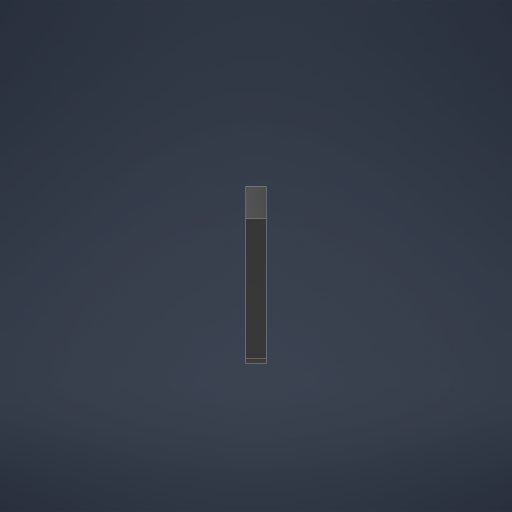
# Autodesk Inventor part: CarbonConnectorStab
Saved by Autodesk Inventor 2023 (Build 270158000, 158)
## iProperties
Created: 2023-02-24
Part Number: CarbonConnectorStab
Material: Generic
Document SubType Name: Modeling
Designer: Elias Braun
Density: 1 g/cm^3
Appearance: Glossy - Black
Author: Elias Braun
Autodesk Inventor part; units mm, degrees
ref_plane "YZ Plane" through (0, 0, 0) normal (1, 0, 0) x (0, 1, 0)
ref_plane "XZ Plane" through (0, 0, 0) normal (0, 1, 0) x (-1, 0, 0)
ref_plane "XY Plane" through (0, 0, 0) normal (0, 0, 1) x (1, 0, 0)
sketch "Sketch3" plane through (0, 0, 0) normal (0, 1, 0) x (-1, 0, 0)
  circle A0 centre (0, 0) radius 110 construction
  arc A1 (43.0581, -98.5) -> (-43.0581, -98.5) centre (0, 0) ccw
  line L0 (0, -107.5) -> (0, -98.5) construction
  line L1 (0, -98.5) -> (0, -73.5) construction
  line L2 (0, -98.5) -> (-43.0581, -98.5) construction
  line L3 (0, -98.5) -> (43.0581, -98.5) construction
  line L4 (43.0581, -98.5) -> (-43.0581, -98.5) construction
  line L5 (-18.0581, -73.5) -> (18.0581, -73.5)
  arc A2 (43.0581, -98.5) -> (18.0581, -73.5) centre (18.0581, -98.5) ccw
  arc A3 (-18.0581, -73.5) -> (-43.0581, -98.5) centre (-18.0581, -98.5) ccw
  line L6 (0, 107.5) -> (0, 97.5) construction
  line L7 (0, 97.5) -> (-22.5, 97.5) construction
  line L8 (-22.5, 97.5) -> (-22.5, 82.5) construction
  line L9 (22.5, 82.5) -> (22.5, 97.5) construction
  line L10 (22.5, 90) -> (-22.5, 90) construction
  line L11 (15, 97.5) -> (-15, 97.5)
  line L12 (-15, 82.5) -> (15, 82.5)
  arc A4 (15, 82.5) -> (15, 97.5) centre (15, 90) ccw
  arc A5 (-15, 97.5) -> (-15, 82.5) centre (-15, 90) ccw
  line L13 (22.5, 82.5) -> (17.5, 82.5) construction
  line L14 (17.5, 82.5) -> (17.5, 77.5) construction
  circle A6 centre (17.5, 77.5) radius 1.6
  circle A7 centre (-17.5, 77.5) radius 1.6
  line L15 (-58.3363, 79.5495) -> (-79.5495, 58.3363)
  arc A8 (-47.7297, 68.9429) -> (-58.3363, 79.5495) centre (-53.033, 74.2462) ccw
  arc A9 (-79.5495, 58.3363) -> (-68.9429, 47.7297) centre (-74.2462, 53.033) ccw
  line L16 (-68.9429, 47.7297) -> (-47.7297, 68.9429)
  circle A10 centre (-67.1751, 42.4264) radius 1.6
  circle A11 centre (-42.4264, 67.1751) radius 1.6
  line L17 (-97.5, 15) -> (-97.5, -15)
  arc A12 (-82.5, 15) -> (-97.5, 15) centre (-90, 15) ccw
  arc A13 (-97.5, -15) -> (-82.5, -15) centre (-90, -15) ccw
  line L18 (-82.5, -15) -> (-82.5, 15)
  circle A14 centre (-77.5, -17.5) radius 1.6
  circle A15 centre (-77.5, 17.5) radius 1.6
  line L19 (-79.5495, -58.3363) -> (-58.3363, -79.5495)
  arc A16 (-68.9429, -47.7297) -> (-79.5495, -58.3363) centre (-74.2462, -53.033) ccw
  arc A17 (-58.3363, -79.5495) -> (-47.7297, -68.9429) centre (-53.033, -74.2462) ccw
  line L20 (-47.7297, -68.9429) -> (-68.9429, -47.7297)
  circle A18 centre (-42.4264, -67.1751) radius 1.6
  circle A19 centre (-67.1751, -42.4264) radius 1.6
  line L21 (-15, -97.5) -> (15, -97.5)
  arc A20 (-15, -82.5) -> (-15, -97.5) centre (-15, -90) ccw
  arc A21 (15, -97.5) -> (15, -82.5) centre (15, -90) ccw
  line L22 (15, -82.5) -> (-15, -82.5)
  circle A22 centre (17.5, -77.5) radius 1.6
  circle A23 centre (-17.5, -77.5) radius 1.6
  line L23 (58.3363, -79.5495) -> (79.5495, -58.3363)
  arc A24 (47.7297, -68.9429) -> (58.3363, -79.5495) centre (53.033, -74.2462) ccw
  arc A25 (79.5495, -58.3363) -> (68.9429, -47.7297) centre (74.2462, -53.033) ccw
  line L24 (68.9429, -47.7297) -> (47.7297, -68.9429)
  circle A26 centre (67.1751, -42.4264) radius 1.6
  circle A27 centre (42.4264, -67.1751) radius 1.6
  line L25 (97.5, -15) -> (97.5, 15)
  arc A28 (82.5, -15) -> (97.5, -15) centre (90, -15) ccw
  arc A29 (97.5, 15) -> (82.5, 15) centre (90, 15) ccw
  line L26 (82.5, 15) -> (82.5, -15)
  circle A30 centre (77.5, 17.5) radius 1.6
  circle A31 centre (77.5, -17.5) radius 1.6
  line L27 (79.5495, 58.3363) -> (58.3363, 79.5495)
  arc A32 (68.9429, 47.7297) -> (79.5495, 58.3363) centre (74.2462, 53.033) ccw
  arc A33 (58.3363, 79.5495) -> (47.7297, 68.9429) centre (53.033, 74.2462) ccw
  line L28 (47.7297, 68.9429) -> (68.9429, 47.7297)
  circle A34 centre (42.4264, 67.1751) radius 1.6
  circle A35 centre (67.1751, 42.4264) radius 1.6
  circle A36 centre (0, 0) radius 110 construction
  arc A37 (43.0581, -98.5) -> (-43.0581, -98.5) centre (0, 0) ccw
  line L29 (0, -107.5) -> (0, -98.5) construction
  line L30 (0, -98.5) -> (0, -73.5) construction
  line L31 (0, -98.5) -> (-43.0581, -98.5) construction
  line L32 (0, -98.5) -> (43.0581, -98.5) construction
  line L33 (43.0581, -98.5) -> (-43.0581, -98.5) construction
  line L34 (-18.0581, -73.5) -> (18.0581, -73.5)
  arc A38 (43.0581, -98.5) -> (18.0581, -73.5) centre (18.0581, -98.5) ccw
  arc A39 (-18.0581, -73.5) -> (-43.0581, -98.5) centre (-18.0581, -98.5) ccw
  line L35 (0, 107.5) -> (0, 97.5) construction
  line L36 (0, 97.5) -> (-22.5, 97.5) construction
  line L37 (-22.5, 97.5) -> (-22.5, 82.5) construction
  line L38 (22.5, 82.5) -> (22.5, 97.5) construction
  line L39 (22.5, 90) -> (-22.5, 90) construction
  line L40 (15, 97.5) -> (-15, 97.5)
  line L41 (-15, 82.5) -> (15, 82.5)
  arc A40 (15, 82.5) -> (15, 97.5) centre (15, 90) ccw
  arc A41 (-15, 97.5) -> (-15, 82.5) centre (-15, 90) ccw
  line L42 (22.5, 82.5) -> (17.5, 82.5) construction
  line L43 (17.5, 82.5) -> (17.5, 77.5) construction
  circle A42 centre (17.5, 77.5) radius 1.6
  circle A43 centre (-17.5, 77.5) radius 1.6
  line L44 (-58.3363, 79.5495) -> (-79.5495, 58.3363)
  arc A44 (-47.7297, 68.9429) -> (-58.3363, 79.5495) centre (-53.033, 74.2462) ccw
  arc A45 (-79.5495, 58.3363) -> (-68.9429, 47.7297) centre (-74.2462, 53.033) ccw
  line L45 (-68.9429, 47.7297) -> (-47.7297, 68.9429)
  circle A46 centre (-67.1751, 42.4264) radius 1.6
  circle A47 centre (-42.4264, 67.1751) radius 1.6
  line L46 (-97.5, 15) -> (-97.5, -15)
  arc A48 (-82.5, 15) -> (-97.5, 15) centre (-90, 15) ccw
  arc A49 (-97.5, -15) -> (-82.5, -15) centre (-90, -15) ccw
  line L47 (-82.5, -15) -> (-82.5, 15)
  circle A50 centre (-77.5, -17.5) radius 1.6
  circle A51 centre (-77.5, 17.5) radius 1.6
  line L48 (-79.5495, -58.3363) -> (-58.3363, -79.5495)
  arc A52 (-68.9429, -47.7297) -> (-79.5495, -58.3363) centre (-74.2462, -53.033) ccw
  arc A53 (-58.3363, -79.5495) -> (-47.7297, -68.9429) centre (-53.033, -74.2462) ccw
  line L49 (-47.7297, -68.9429) -> (-68.9429, -47.7297)
  circle A54 centre (-42.4264, -67.1751) radius 1.6
  circle A55 centre (-67.1751, -42.4264) radius 1.6
  line L50 (-15, -97.5) -> (15, -97.5)
  arc A56 (-15, -82.5) -> (-15, -97.5) centre (-15, -90) ccw
  arc A57 (15, -97.5) -> (15, -82.5) centre (15, -90) ccw
  line L51 (15, -82.5) -> (-15, -82.5)
  circle A58 centre (17.5, -77.5) radius 1.6
  circle A59 centre (-17.5, -77.5) radius 1.6
  line L52 (58.3363, -79.5495) -> (79.5495, -58.3363)
  arc A60 (47.7297, -68.9429) -> (58.3363, -79.5495) centre (53.033, -74.2462) ccw
  arc A61 (79.5495, -58.3363) -> (68.9429, -47.7297) centre (74.2462, -53.033) ccw
  line L53 (68.9429, -47.7297) -> (47.7297, -68.9429)
  circle A62 centre (67.1751, -42.4264) radius 1.6
  circle A63 centre (42.4264, -67.1751) radius 1.6
  line L54 (97.5, -15) -> (97.5, 15)
  arc A64 (82.5, -15) -> (97.5, -15) centre (90, -15) ccw
  arc A65 (97.5, 15) -> (82.5, 15) centre (90, 15) ccw
  line L55 (82.5, 15) -> (82.5, -15)
  circle A66 centre (77.5, 17.5) radius 1.6
  circle A67 centre (77.5, -17.5) radius 1.6
  line L56 (79.5495, 58.3363) -> (58.3363, 79.5495)
  arc A68 (68.9429, 47.7297) -> (79.5495, 58.3363) centre (74.2462, 53.033) ccw
  arc A69 (58.3363, 79.5495) -> (47.7297, 68.9429) centre (53.033, 74.2462) ccw
  line L57 (47.7297, 68.9429) -> (68.9429, 47.7297)
  circle A70 centre (42.4264, 67.1751) radius 1.6
  circle A71 centre (67.1751, 42.4264) radius 1.6
  line L58 (67.1751, -42.4264) -> (54.8008, -54.8008) construction
  line L59 (54.8008, -54.8008) -> (53.3866, -56.215) construction
  line L60 (53.3866, -56.215) -> (52.3259, -57.2756) construction
  line L61 (47.7297, -54.8008) -> (54.8008, -61.8718)
  line L62 (54.8008, -61.8718) -> (56.9221, -59.7505)
  line L63 (56.9221, -59.7505) -> (49.851, -52.6795)
  line L64 (49.851, -52.6795) -> (47.7297, -54.8008)
  line L65 (47.7297, -54.8008) -> (56.9221, -59.7505) construction
  line L66 (54.8008, -61.8718) -> (49.851, -52.6795) construction
  line L67 (54.8008, -54.8008) -> (53.7401, -53.7401) construction
  line L68 (59.7505, -56.9221) -> (52.6795, -49.851)
  line L69 (54.8008, -47.7297) -> (61.8718, -54.8008)
  line L70 (52.6795, -49.851) -> (54.8008, -47.7297)
  line L71 (58.9727, -57.6999) -> (51.9016, -50.6288)
  line L72 (51.9016, -50.6288) -> (50.6288, -51.9016)
  line L73 (50.6288, -51.9016) -> (57.6999, -58.9727)
  line L74 (57.6999, -58.9727) -> (58.9727, -57.6999)
  line L75 (58.9727, -57.6999) -> (50.6288, -51.9016) construction
  line L76 (51.9016, -50.6288) -> (57.6999, -58.9727) construction
  point P0 (0, 90)
  point P1 (-45.9619, 70.7107)
  point P2 (-82.5, 17.5)
  point P3 (-70.7107, -45.9619)
  point P4 (-17.5, -82.5)
  point P5 (45.9619, -70.7107)
  point P6 (82.5, -17.5)
  point P7 (70.7107, 45.9619)
  point P8 (0, 90)
  point P9 (-45.9619, 70.7107)
  point P10 (-82.5, 17.5)
  point P11 (-70.7107, -45.9619)
  point P12 (-17.5, -82.5)
  point P13 (45.9619, -70.7107)
  point P14 (82.5, -17.5)
  point P15 (70.7107, 45.9619)
  point P16 (45.4935, 0)
  point P17 (26.7551, 33.8262)
  point P18 (-26.7551, 33.8262)
  point P19 (-33.8262, 26.7551)
  point P20 (-33.8262, -26.7551)
  point P21 (-26.7551, -33.8262)
  point P22 (26.7551, -33.8262)
  point P23 (33.8262, -26.7551)
  point P24 (33.8262, 26.7551)
  dimension "d9" = 220
  dimension "d10" = 215
  dimension "d11" = 9
  dimension "d12" = 25
  dimension "d13" = 10
  dimension "d14" = 22.5
  dimension "d15" = 15
  dimension "d16" = 45
  dimension "d17" = 5
  dimension "d18" = 5
  dimension "d19" = 3.2
  dimension "d20" = 86.1162
  dimension "d21" = 45
  dimension "d22" = 360
  dimension "d23" = 220
  dimension "d24" = 215
  dimension "d25" = 9
  dimension "d26" = 25
  dimension "d27" = 10
  dimension "d28" = 22.5
  dimension "d29" = 15
  dimension "d30" = 45
  dimension "d31" = 5
  dimension "d32" = 5
  dimension "d33" = 3.2
  dimension "d34" = 86.1162
  dimension "d35" = 45
  dimension "d36" = 360
  dimension "d37" = 17.5
  dimension "d38" = 2
  dimension "d39" = 1.5
  dimension "d40" = 1.8
  constraints: 162 end point, 86 point on circle, 72 centre point, 30 point on line, 12 midpoint, 12 tangent, 6 coincident, 6 parallel, 6 symmetric about line, 6 vertical, 4 horizontal, 3 perpendicular, 2 collinear, 244 other
  measures "d9" diameter of A0
  measures "d10" diameter of A1
  measures "d11" distance of L0.start L0.end
  measures "d12" distance of L0.end L1.end
  measures "d13" distance of L6.start L6.end
  measures "d14" distance of L6.end L7.end
  measures "d15" distance of L7.end L8.end
  measures "d16" distance of L8.end L9.start
  measures "d17" distance of L9.start L13.end
  measures "d18" distance of L13.end L14.end
  measures "d19" diameter of A6
  measures "d20" distance of L3.end L2.end
  measures "d21" distance of L10.start L10.end
  measures "d23" diameter of A36
  measures "d24" diameter of A37
  measures "d25" distance of L29.start L29.end
  measures "d26" distance of L29.end L30.end
  measures "d27" distance of L35.start L35.end
  measures "d28" distance of L35.end L36.end
  measures "d29" distance of L36.end L37.end
  measures "d30" distance of L37.end L38.start
  measures "d31" distance of L38.start L42.end
  measures "d32" distance of L42.end L43.end
  measures "d33" diameter of A42
  measures "d34" distance of L32.end L31.end
  measures "d35" distance of L39.start L39.end
  measures "d37" distance of L58.start L58.end
  measures "d38" distance of L58.end L59.end
  measures "d39" distance of L59.end L60.end
  measures "d40" distance of L72.end L71.end
extrude "Extrusion2" add sketch "Sketch3" along normal blind 4.5 contours L73 L72 L71 L24
sketch "Sketch4" plane through (-51.9016, 0, -50.6288) normal (-0.7071068, 0, 0.7071068) x (0.7071068, 0, 0.7071068)
  line L0 (0, 4.5) -> (-10, 4.5) construction
  line L1 (0, 0) -> (-10, 0) construction
  line L2 (-10, 4.5) -> (0, 0) construction
  line L3 (-5, 2.25) -> (-7.5, 2.25) construction
  line L4 (-10, 0) -> (-10, 4.5) construction
  line L5 (-5, 2.25) -> (-5, 3.2445) construction
  circle A0 centre (-7.5, 2.25) radius 1.1
  circle A1 centre (-2.5, 2.25) radius 1.1
  point P0 (72.5, 0)
  dimension "d43" = 2.5
  dimension "d44" = 2.2
  constraints: 6 end point, 2 centre point, 1 coincident, 1 midpoint, 1 perpendicular, 1 symmetric about line, 1 vertical, 1 other
  measures "d43" distance of L3.start L3.end
  measures "d44" diameter of A0
extrude "Extrusion3" cut sketch "Sketch4" against normal blind 4.5
ref_plane "Work Plane2" through (0, 19.5, 0) normal (0, 1, 0) x (1, 0, 0)
sketch "Sketch5" plane through (0, 19.5, 0) normal (0, 1, 0) x (1, 0, 0)
  circle A0 centre (0, 0) radius 110 construction
  arc A1 (43.0581, -98.5) -> (-43.0581, -98.5) centre (0, 0) ccw
  line L0 (0, -107.5) -> (0, -98.5) construction
  line L1 (0, -98.5) -> (0, -73.5) construction
  line L2 (0, -98.5) -> (-43.0581, -98.5) construction
  line L3 (0, -98.5) -> (43.0581, -98.5) construction
  line L4 (43.0581, -98.5) -> (-43.0581, -98.5) construction
  line L5 (-18.0581, -73.5) -> (18.0581, -73.5)
  arc A2 (43.0581, -98.5) -> (18.0581, -73.5) centre (18.0581, -98.5) ccw
  arc A3 (-18.0581, -73.5) -> (-43.0581, -98.5) centre (-18.0581, -98.5) ccw
  line L6 (0, 107.5) -> (0, 97.5) construction
  line L7 (0, 97.5) -> (-22.5, 97.5) construction
  line L8 (-22.5, 97.5) -> (-22.5, 82.5) construction
  line L9 (22.5, 82.5) -> (22.5, 97.5) construction
  line L10 (22.5, 90) -> (-22.5, 90) construction
  line L11 (15, 97.5) -> (-15, 97.5)
  line L12 (-15, 82.5) -> (15, 82.5)
  arc A4 (15, 82.5) -> (15, 97.5) centre (15, 90) ccw
  arc A5 (-15, 97.5) -> (-15, 82.5) centre (-15, 90) ccw
  line L13 (22.5, 82.5) -> (17.5, 82.5) construction
  line L14 (17.5, 82.5) -> (17.5, 77.5) construction
  circle A6 centre (17.5, 77.5) radius 1.6
  circle A7 centre (-17.5, 77.5) radius 1.6
  line L15 (-58.3363, 79.5495) -> (-79.5495, 58.3363)
  arc A8 (-47.7297, 68.9429) -> (-58.3363, 79.5495) centre (-53.033, 74.2462) ccw
  arc A9 (-79.5495, 58.3363) -> (-68.9429, 47.7297) centre (-74.2462, 53.033) ccw
  line L16 (-68.9429, 47.7297) -> (-47.7297, 68.9429)
  circle A10 centre (-67.1751, 42.4264) radius 1.6
  circle A11 centre (-42.4264, 67.1751) radius 1.6
  line L17 (-97.5, 15) -> (-97.5, -15)
  arc A12 (-82.5, 15) -> (-97.5, 15) centre (-90, 15) ccw
  arc A13 (-97.5, -15) -> (-82.5, -15) centre (-90, -15) ccw
  line L18 (-82.5, -15) -> (-82.5, 15)
  circle A14 centre (-77.5, -17.5) radius 1.6
  circle A15 centre (-77.5, 17.5) radius 1.6
  line L19 (-79.5495, -58.3363) -> (-58.3363, -79.5495)
  arc A16 (-68.9429, -47.7297) -> (-79.5495, -58.3363) centre (-74.2462, -53.033) ccw
  arc A17 (-58.3363, -79.5495) -> (-47.7297, -68.9429) centre (-53.033, -74.2462) ccw
  line L20 (-47.7297, -68.9429) -> (-68.9429, -47.7297)
  circle A18 centre (-42.4264, -67.1751) radius 1.6
  circle A19 centre (-67.1751, -42.4264) radius 1.6
  line L21 (-15, -97.5) -> (15, -97.5)
  arc A20 (-15, -82.5) -> (-15, -97.5) centre (-15, -90) ccw
  arc A21 (15, -97.5) -> (15, -82.5) centre (15, -90) ccw
  line L22 (15, -82.5) -> (-15, -82.5)
  circle A22 centre (17.5, -77.5) radius 1.6
  circle A23 centre (-17.5, -77.5) radius 1.6
  line L23 (58.3363, -79.5495) -> (79.5495, -58.3363)
  arc A24 (47.7297, -68.9429) -> (58.3363, -79.5495) centre (53.033, -74.2462) ccw
  arc A25 (79.5495, -58.3363) -> (68.9429, -47.7297) centre (74.2462, -53.033) ccw
  line L24 (68.9429, -47.7297) -> (47.7297, -68.9429)
  circle A26 centre (67.1751, -42.4264) radius 1.6
  circle A27 centre (42.4264, -67.1751) radius 1.6
  line L25 (97.5, -15) -> (97.5, 15)
  arc A28 (82.5, -15) -> (97.5, -15) centre (90, -15) ccw
  arc A29 (97.5, 15) -> (82.5, 15) centre (90, 15) ccw
  line L26 (82.5, 15) -> (82.5, -15)
  circle A30 centre (77.5, 17.5) radius 1.6
  circle A31 centre (77.5, -17.5) radius 1.6
  line L27 (79.5495, 58.3363) -> (58.3363, 79.5495)
  arc A32 (68.9429, 47.7297) -> (79.5495, 58.3363) centre (74.2462, 53.033) ccw
  arc A33 (58.3363, 79.5495) -> (47.7297, 68.9429) centre (53.033, 74.2462) ccw
  line L28 (47.7297, 68.9429) -> (68.9429, 47.7297)
  circle A34 centre (42.4264, 67.1751) radius 1.6
  circle A35 centre (67.1751, 42.4264) radius 1.6
  circle A36 centre (0, 0) radius 110 construction
  arc A37 (43.0581, -98.5) -> (-43.0581, -98.5) centre (0, 0) ccw
  line L29 (0, -107.5) -> (0, -98.5) construction
  line L30 (0, -98.5) -> (0, -73.5) construction
  line L31 (0, -98.5) -> (-43.0581, -98.5) construction
  line L32 (0, -98.5) -> (43.0581, -98.5) construction
  line L33 (43.0581, -98.5) -> (-43.0581, -98.5) construction
  line L34 (-18.0581, -73.5) -> (18.0581, -73.5)
  arc A38 (43.0581, -98.5) -> (18.0581, -73.5) centre (18.0581, -98.5) ccw
  arc A39 (-18.0581, -73.5) -> (-43.0581, -98.5) centre (-18.0581, -98.5) ccw
  line L35 (0, 107.5) -> (0, 97.5) construction
  line L36 (0, 97.5) -> (-22.5, 97.5) construction
  line L37 (-22.5, 97.5) -> (-22.5, 82.5) construction
  line L38 (22.5, 82.5) -> (22.5, 97.5) construction
  line L39 (22.5, 90) -> (-22.5, 90) construction
  line L40 (15, 97.5) -> (-15, 97.5)
  line L41 (-15, 82.5) -> (15, 82.5)
  arc A40 (15, 82.5) -> (15, 97.5) centre (15, 90) ccw
  arc A41 (-15, 97.5) -> (-15, 82.5) centre (-15, 90) ccw
  line L42 (22.5, 82.5) -> (17.5, 82.5) construction
  line L43 (17.5, 82.5) -> (17.5, 77.5) construction
  circle A42 centre (17.5, 77.5) radius 1.6
  circle A43 centre (-17.5, 77.5) radius 1.6
  line L44 (-58.3363, 79.5495) -> (-79.5495, 58.3363)
  arc A44 (-47.7297, 68.9429) -> (-58.3363, 79.5495) centre (-53.033, 74.2462) ccw
  arc A45 (-79.5495, 58.3363) -> (-68.9429, 47.7297) centre (-74.2462, 53.033) ccw
  line L45 (-68.9429, 47.7297) -> (-47.7297, 68.9429)
  circle A46 centre (-67.1751, 42.4264) radius 1.6
  circle A47 centre (-42.4264, 67.1751) radius 1.6
  line L46 (-97.5, 15) -> (-97.5, -15)
  arc A48 (-82.5, 15) -> (-97.5, 15) centre (-90, 15) ccw
  arc A49 (-97.5, -15) -> (-82.5, -15) centre (-90, -15) ccw
  line L47 (-82.5, -15) -> (-82.5, 15)
  circle A50 centre (-77.5, -17.5) radius 1.6
  circle A51 centre (-77.5, 17.5) radius 1.6
  line L48 (-79.5495, -58.3363) -> (-58.3363, -79.5495)
  arc A52 (-68.9429, -47.7297) -> (-79.5495, -58.3363) centre (-74.2462, -53.033) ccw
  arc A53 (-58.3363, -79.5495) -> (-47.7297, -68.9429) centre (-53.033, -74.2462) ccw
  line L49 (-47.7297, -68.9429) -> (-68.9429, -47.7297)
  circle A54 centre (-42.4264, -67.1751) radius 1.6
  circle A55 centre (-67.1751, -42.4264) radius 1.6
  line L50 (-15, -97.5) -> (15, -97.5)
  arc A56 (-15, -82.5) -> (-15, -97.5) centre (-15, -90) ccw
  arc A57 (15, -97.5) -> (15, -82.5) centre (15, -90) ccw
  line L51 (15, -82.5) -> (-15, -82.5)
  circle A58 centre (17.5, -77.5) radius 1.6
  circle A59 centre (-17.5, -77.5) radius 1.6
  line L52 (58.3363, -79.5495) -> (79.5495, -58.3363)
  arc A60 (47.7297, -68.9429) -> (58.3363, -79.5495) centre (53.033, -74.2462) ccw
  arc A61 (79.5495, -58.3363) -> (68.9429, -47.7297) centre (74.2462, -53.033) ccw
  line L53 (68.9429, -47.7297) -> (47.7297, -68.9429)
  circle A62 centre (67.1751, -42.4264) radius 1.6
  circle A63 centre (42.4264, -67.1751) radius 1.6
  line L54 (97.5, -15) -> (97.5, 15)
  arc A64 (82.5, -15) -> (97.5, -15) centre (90, -15) ccw
  arc A65 (97.5, 15) -> (82.5, 15) centre (90, 15) ccw
  line L55 (82.5, 15) -> (82.5, -15)
  circle A66 centre (77.5, 17.5) radius 1.6
  circle A67 centre (77.5, -17.5) radius 1.6
  line L56 (79.5495, 58.3363) -> (58.3363, 79.5495)
  arc A68 (68.9429, 47.7297) -> (79.5495, 58.3363) centre (74.2462, 53.033) ccw
  arc A69 (58.3363, 79.5495) -> (47.7297, 68.9429) centre (53.033, 74.2462) ccw
  line L57 (47.7297, 68.9429) -> (68.9429, 47.7297)
  circle A70 centre (42.4264, 67.1751) radius 1.6
  circle A71 centre (67.1751, 42.4264) radius 1.6
  line L58 (67.1751, -42.4264) -> (54.8008, -54.8008) construction
  line L59 (54.8008, -54.8008) -> (53.3866, -56.215) construction
  line L60 (53.3866, -56.215) -> (52.3259, -57.2756) construction
  line L61 (47.7297, -54.8008) -> (54.8008, -61.8718)
  line L62 (54.8008, -61.8718) -> (56.9221, -59.7505)
  line L63 (56.9221, -59.7505) -> (49.851, -52.6795)
  line L64 (49.851, -52.6795) -> (47.7297, -54.8008)
  line L65 (47.7297, -54.8008) -> (56.9221, -59.7505) construction
  line L66 (54.8008, -61.8718) -> (49.851, -52.6795) construction
  line L67 (54.8008, -54.8008) -> (53.7401, -53.7401) construction
  line L68 (59.7505, -56.9221) -> (52.6795, -49.851)
  line L69 (54.8008, -47.7297) -> (61.8718, -54.8008)
  line L70 (52.6795, -49.851) -> (54.8008, -47.7297)
  circle A72 centre (0, 0) radius 75 construction
  circle A73 centre (0, 0) radius 55 construction
  line L71 (-51.9016, 50.6288) -> (-50.6288, 51.9016) construction
  line L72 (-51.2652, 51.2652) -> (-37.8825, 37.8825) construction
  line L73 (-41.295, 40.0222) -> (-37.7595, 36.4867)
  line L74 (-37.7595, 36.4867) -> (-36.4867, 37.7595)
  line L75 (-36.4867, 37.7595) -> (-40.0222, 41.295)
  line L76 (-40.0222, 41.295) -> (-41.295, 40.0222)
  line L77 (-41.295, 40.0222) -> (-36.4867, 37.7595) construction
  line L78 (-37.7595, 36.4867) -> (-40.0222, 41.295) construction
  point P0 (0, 90)
  point P1 (-45.9619, 70.7107)
  point P2 (-82.5, 17.5)
  point P3 (-70.7107, -45.9619)
  point P4 (-17.5, -82.5)
  point P5 (45.9619, -70.7107)
  point P6 (82.5, -17.5)
  point P7 (70.7107, 45.9619)
  point P8 (0, 90)
  point P9 (-45.9619, 70.7107)
  point P10 (-82.5, 17.5)
  point P11 (-70.7107, -45.9619)
  point P12 (-17.5, -82.5)
  point P13 (45.9619, -70.7107)
  point P14 (82.5, -17.5)
  point P15 (70.7107, 45.9619)
  point P16 (45.4935, 0)
  point P17 (26.7551, 33.8262)
  point P18 (-26.7551, 33.8262)
  point P19 (-33.8262, 26.7551)
  point P20 (-33.8262, -26.7551)
  point P21 (-26.7551, -33.8262)
  point P22 (26.7551, -33.8262)
  point P23 (33.8262, -26.7551)
  point P24 (33.8262, 26.7551)
  point P25 (-38.8909, 38.8909)
  dimension "d84" = 110
  dimension "d52" = 220
  dimension "d53" = 215
  dimension "d54" = 9
  dimension "d55" = 25
  dimension "d56" = 10
  dimension "d57" = 22.5
  dimension "d58" = 15
  dimension "d59" = 45
  dimension "d60" = 5
  dimension "d61" = 5
  dimension "d62" = 3.2
  dimension "d63" = 86.1162
  dimension "d64" = 45
  dimension "d65" = 360
  dimension "d66" = 220
  dimension "d67" = 215
  dimension "d68" = 9
  dimension "d69" = 25
  dimension "d70" = 10
  dimension "d71" = 22.5
  dimension "d72" = 15
  dimension "d73" = 45
  dimension "d74" = 5
  dimension "d75" = 5
  dimension "d76" = 3.2
  dimension "d77" = 86.1162
  dimension "d78" = 45
  dimension "d79" = 360
  dimension "d80" = 17.5
  dimension "d81" = 2
  dimension "d82" = 1.5
  dimension "d83" = 150
  dimension "d85" = 5
  constraints: 164 end point, 86 point on circle, 73 centre point, 31 point on line, 13 midpoint, 12 tangent, 8 coincident, 6 parallel, 6 symmetric about line, 6 vertical, 4 horizontal, 4 perpendicular, 2 collinear, 247 other
  measures "d52" diameter of A0
  measures "d53" diameter of A1
  measures "d54" distance of L0.start L0.end
  measures "d55" distance of L0.end L1.end
  measures "d56" distance of L6.start L6.end
  measures "d57" distance of L6.end L7.end
  measures "d58" distance of L7.end L8.end
  measures "d59" distance of L8.end L9.start
  measures "d60" distance of L9.start L13.end
  measures "d61" distance of L13.end L14.end
  measures "d62" diameter of A6
  measures "d63" distance of L3.end L2.end
  measures "d64" distance of L10.start L10.end
  measures "d66" diameter of A36
  measures "d67" diameter of A37
  measures "d68" distance of L29.start L29.end
  measures "d69" distance of L29.end L30.end
  measures "d70" distance of L35.start L35.end
  measures "d71" distance of L35.end L36.end
  measures "d72" distance of L36.end L37.end
  measures "d73" distance of L37.end L38.start
  measures "d74" distance of L38.start L42.end
  measures "d75" distance of L42.end L43.end
  measures "d76" diameter of A42
  measures "d77" distance of L32.end L31.end
  measures "d78" distance of L39.start L39.end
  measures "d80" distance of L58.start L58.end
  measures "d81" distance of L58.end L59.end
  measures "d82" distance of L59.end L60.end
  measures "d83" diameter of A72
  measures "d85" distance of L73.start L73.end
extrude "Extrusion4" add sketch "Sketch5" along normal mid plane 12 contours L76 L75 L74 L73
ref_plane "Work Plane4" through (-58.9727, 4.5, -57.6999) normal (-0.7071068, 0, 0.7071068) x (0.7071068, 0, 0.7071068)
sketch "Sketch8" plane through (-58.9727, 4.5, -57.6999) normal (-0.7071068, 0, 0.7071068) x (0.7071068, 0, 0.7071068)
  line L0 (10, 0) -> (0, 0) projected
  line L1 (10, -4.5) -> (0, -4.5) projected
  line L2 (10, 0) -> (10, -4.5)
  line L3 (25, 9) -> (30, 9) projected
  line L4 (30, 9) -> (25, 9)
  line L5 (10, -4.5) -> (30, 9)
  line L6 (10, -4.5) -> (17.9179, -4.5) construction
  line L7 (10, 0) -> (12.3461, 0) construction
  line L8 (10, 0) -> (25, 10.125)
  line L9 (10, 0) -> (30, 0) construction
  line L10 (25, 9) -> (25, 21) projected
  line L11 (25, 10.125) -> (25, 9)
  line L12 (25, 9) -> (30, 9)
  point P0 (82.5, -4.5)
  dimension "d92" = 34.019
  dimension "d94" = 34.019
  constraints: 18 end point, 2 horizontal, 2 vertical, 1 collinear, 1 perpendicular, 1 point on line
  measures "d92" angle of L5 L6
  measures "d94" angle of L9 L8
extrude "Extrusion6" add sketch "Sketch8" against normal blind 1.8
fillet "Fillet1" radius 1 4 edges at (-51.2652, 4.5, -51.2652) (-40.6586, 14.625, -40.6586) (-51.2652, 0, -51.2652) (-37.1231, 13.5, -37.1231)
sketch "Sketch9" plane through (0, 25.5, 0) normal (0, 1, 0) x (1, 0, 0)
  line L0 (-36.4867, 37.7595) -> (-40.0222, 41.295) projected
  line L1 (-36.4867, 37.7595) -> (-37.7595, 36.4867)
  line L2 (-51.7223, 50.4496) -> (-38.071, 36.7982) projected
  line L3 (-37.7595, 36.4867) -> (-41.295, 40.0222)
  line L4 (-41.295, 40.0222) -> (-40.0222, 41.295) projected
  line L5 (-40.0222, 41.295) -> (-41.295, 40.0222)
  line L6 (-41.295, 40.0222) -> (-40.0222, 41.295)
  line L7 (-36.7982, 38.071) -> (-50.4496, 51.7223) projected
  line L8 (-40.0222, 41.295) -> (-36.4867, 37.7595)
  point P0 (0, 0)
  constraints: 10 end point, 3 perpendicular, 1 collinear, 1 point on line
extrude "Extrusion7" add sketch "Sketch9" along normal blind 4
sketch "Sketch10" plane through (-58.9727, 0, -57.6999) normal (-0.7071068, 0, 0.7071068) x (0.7071068, 0, 0.7071068)
  line L0 (25, 29.5) -> (30, 29.5) projected
  line L1 (27.5, 29.5) -> (27.5, 26.5) construction
  line L2 (27.5, 26.5) -> (27.5, 20.5) construction
  circle A0 centre (27.5, 26.5) radius 1.1
  circle A1 centre (27.5, 20.5) radius 1.1
  point P0 (82.5, 0)
  dimension "d100" = 3
  dimension "d101" = 6
  dimension "d102" = 2.2
  dimension "d103" = 2.2
  constraints: 4 end point, 2 centre point, 2 coincident, 2 vertical, 1 midpoint
  measures "d100" distance of L1.start L1.end
  measures "d101" distance of L1.end L2.end
  measures "d102" diameter of A0
  measures "d103" diameter of A1
extrude "Extrusion8" cut sketch "Sketch10" against normal blind 4
body "Solid2"
